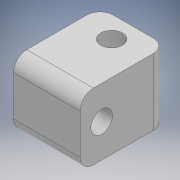
# Autodesk Inventor part: CardanJoint
Saved by Autodesk Inventor 2018 (Build 220112000, 112)
## iProperties
Created: 2020-03-23
Part Number: CardanJoint
Material: Generic
Document SubType Name: Modeling
Designer: technik
Density: 1 g/cm^3
Appearance: Default
Mass: 1.05557 g
Surface Area: 8.22794 cm^2
Volume: 1.05557 cm^3
Author: technik
Autodesk Inventor part; units mm, degrees
ref_plane "YZ Plane" through (0, 0, 0) normal (1, 0, 0) x (0, 1, 0)
ref_plane "XZ Plane" through (0, 0, 0) normal (0, 1, 0) x (-1, 0, 0)
ref_plane "XY Plane" through (0, 0, 0) normal (0, 0, 1) x (1, 0, 0)
sketch "Sketch7" plane through (0, 0, 0) normal (0, 0, 1) x (1, 0, 0)
  line L0 (-5, 6.5) -> (5, 6.5)
  line L1 (5, 6.5) -> (5, -6.5)
  line L2 (5, -6.5) -> (-5, -6.5)
  line L3 (-5, -6.5) -> (-5, 6.5)
  line L4 (0, 6.5) -> (0, -6.5)
  line L5 (-5, 0) -> (5, 0)
  point P0 (0, 0)
  point P1 (0, 0)
  dimension "d14" = 10
  dimension "d15" = 13
  constraints: 12 end point, 5 midpoint, 2 parallel, 1 coincident, 1 horizontal, 1 perpendicular
  measures "d14" distance of L1.end L2.end
  measures "d15" distance of L0.end L1.end
extrude "Extrusion4" add sketch "Sketch7" along normal blind 10
sketch "Sketch8" plane through (5, -6.5, 0) normal (1, 0, 0) x (0, 0, -1)
  line L0 (0, 13) -> (-10, 13) projected
  line L1 (-5, 13) -> (-5, 0)
  line L2 (0, 0) -> (-10, 0) projected
  line L3 (0, 6.5) -> (-10, 6.5)
  line L4 (-10, 13) -> (-10, 0) projected
  line L5 (0, 0) -> (-10, 0) projected
  circle A0 centre (-5, 3.25) radius 1.625
  dimension "d18" = 3.25
  dimension "d27" = 3.25
  constraints: 4 end point, 3 midpoint, 1 centre point, 1 point on line
  measures "d18" diameter of A0
  measures "d27" distance from line of L3 A0.centre
extrude "Extrusion5" cut sketch "Sketch8" against normal through all contours A0 L1 | L1 A0
sketch "Sketch9" plane through (0, 0, 10) normal (0, 0, 1) x (1, 0, 0)
  line L0 (-5, 6.5) -> (-5, -6.5) projected
  line L1 (-5, 0) -> (5, 0)
  line L2 (5, -6.5) -> (5, 6.5) projected
  line L3 (0, 0) -> (0, 1.625)
  line L4 (5, 6.5) -> (-5, 6.5) projected
  circle A0 centre (0, 3.25) radius 1.625
  dimension "d22" = 3.25
  dimension "d28" = 3.25
  constraints: 4 end point, 2 midpoint, 1 point on line, 1 vertical alignment, 2 other
  measures "d28" distance from line of L1 point (0, 3.25)
extrude "Extrusion6" cut sketch "Sketch9" against normal through all contours A0
fillet "Fillet2" radius 2 4 edges at (5, 6.5, 5) (-5, 6.5, 5) (0, -6.5, 10) (0, -6.5, 0)
body "Solid3"
